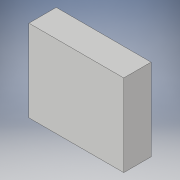
# Autodesk Inventor part: supportBlock
Saved by Autodesk Inventor 2018.2 (Build 222227000, 227)
## iProperties
Created: 2018-02-11
Part Number: supportBlock
Material: Generic
Document SubType Name: Modeling
Designer: steele
Density: 1 g/cm^3
Appearance: Default
Author: steele
Autodesk Inventor part; units mm, degrees
ref_plane "YZ Plane" through (0, 0, 0) normal (1, 0, 0) x (0, 1, 0)
ref_plane "XZ Plane" through (0, 0, 0) normal (0, 1, 0) x (-1, 0, 0)
ref_plane "XY Plane" through (0, 0, 0) normal (0, 0, 1) x (1, 0, 0)
sketch "Sketch1" plane through (0, 0, 0) normal (0, 0, 1) x (1, 0, 0)
  line L0 (-44.069, -38.1) -> (44.069, -38.1)
  line L1 (44.069, -38.1) -> (44.069, 38.1)
  line L2 (44.069, 38.1) -> (-44.069, 38.1)
  line L3 (-44.069, 38.1) -> (-44.069, -38.1)
  line L4 (-44.069, -38.1) -> (44.069, 38.1) construction
  line L5 (44.069, -38.1) -> (-44.069, 38.1) construction
  point P0 (0, 0)
  dimension "d0" = 88.138
  dimension "d1" = 76.2
  constraints: 12 end point, 2 midpoint, 2 parallel, 1 horizontal, 1 perpendicular
  measures "d0" distance of L0.start L0.end
  measures "d1" distance of L1.end L0.end
extrude "Extrusion1" add sketch "Sketch1" against normal blind 25.4
body "Solid1"
